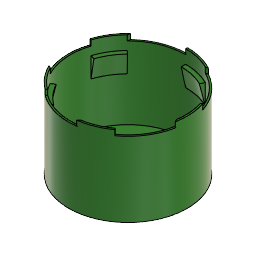
frame-base (Autodesk Fusion 360 design; units mm, degrees)
part number: 2026-06-05-14-14-42-148
Autodesk Fusion 360 part; units mm, degrees
note: some values were not read from the file. Set by a fixed rule: which sketch regions a step uses.
sketch "Sketch1" plane through (0, 0, 0) normal (0, 0, 1) x (1, 0, 0)
  circle A0 centre (0, 0) radius 65.5
  circle A1 centre (0, 0) radius 67.5
  line L0 (0, 0) -> (0, 65.5)
  line L1 (0, 0) -> (29.226, 58.6182)
  line L2 (29.226, 58.6182) -> (32.4791, 59.1723)
  line L3 (0, 65.5) -> (0, 67.5)
  line L4 (-62.2942, 20.2406) -> (-64.1963, 20.8586)
  line L5 (-46.7179, 45.9096) -> (-46.2396, 49.1747)
  line L6 (-38.4999, -52.9906) -> (-39.6755, -54.6086)
  line L7 (-58.0992, -30.2445) -> (-61.0567, -28.7806)
  line L8 (38.4999, -52.9906) -> (39.6755, -54.6086)
  line L9 (10.8106, -64.6017) -> (8.5044, -66.9621)
  line L10 (62.2942, 20.2406) -> (64.1963, 20.8586)
  line L11 (64.7805, -9.6815) -> (66.3128, -12.6042)
  line L12 (0, 60.5) -> (0, 65.5)
  line L13 (26.995, 54.1435) -> (29.226, 58.6182)
  arc A2 (26.995, 54.1435) -> (0, 60.5) centre (0, 0) ccw
  line L14 (-57.5389, 18.6955) -> (-62.2942, 20.2406)
  arc A3 (-43.1517, 42.405) -> (-57.5389, 18.6955) centre (0, 0) ccw
  line L15 (-43.1517, 42.405) -> (-46.7179, 45.9096)
  line L16 (-35.561, -48.9455) -> (-38.4999, -52.9906)
  arc A4 (-53.6642, -27.9358) -> (-35.561, -48.9455) centre (0, 0) ccw
  line L17 (-53.6642, -27.9358) -> (-58.0992, -30.2445)
  line L18 (35.561, -48.9455) -> (38.4999, -52.9906)
  arc A5 (9.9854, -59.6703) -> (35.561, -48.9455) centre (0, 0) ccw
  line L19 (9.9854, -59.6703) -> (10.8106, -64.6017)
  line L20 (57.5389, 18.6955) -> (62.2942, 20.2406)
  arc A6 (59.8355, -8.9425) -> (57.5389, 18.6955) centre (0, 0) ccw
  line L21 (59.8355, -8.9425) -> (64.7805, -9.6815)
  dimension "d1" = 131
  dimension "d2" = 135
  dimension "d3" = 26.5
  dimension "d4" = 3.3
  dimension "d8" = 360
  dimension "d13" = 121
  dimension "d15" = 360
  constraint coincident A0.centre A1.centre
  constraint concentric A0 A1
  constraint vertical L0
  constraint coincident A0 L1.end
  constraint coincident A0 L0.end
  constraint coincident A1 L2.end
  constraint coincident A1 L3.end
  constraint parallel L0 L3
  constraint concentric A0 A2
  constraint coincident L0 L12.start
  constraint coincident L1 L13.start
  measures "d1" diameter of A0
  measures "d2" diameter of A1
  measures "d3" angle of L0 L1
  measures "d4" distance of L1.end L2.end
  measures "d13" diameter of A2
extrude "Extrude1" add sketch "Sketch1" along normal blind 2.5 contours A0 L20 A6 L21 | A0 L0 L1 L12 L13 L14 A3 L15 L16 A4 L17 L18 A5 L19 L20 A6 L21 | A0 L0 L1 L12 L13 A2 | A0 L18 A5 L19 | L0 L1 A2 | A0 L14 A3 L15 | A0 L16 A4 L17 makes body 1
extrude "Extrude2" add sketch "Sketch1" along normal blind 85 contours A0 A1 L2 L10 | A0 A1 L8 L11 | A0 A1 L3 L5 | A0 A1 L6 L9 | A0 A1 L4 L7 bodies 1
extrude "Extrude3" add sketch "Sketch1" along normal blind 91 contours A0 A1 L10 L11 | A0 A1 L2 L3 | A0 A1 L8 L9 | A0 A1 L4 L5 | A0 A1 L6 L7 bodies 1
extrude "Extrude4" add sketch "Sketch1" along normal blind 23 from surface at 52.5 separate body contours A0 L20 A6 L21 | A0 L0 L1 L12 L13 A2 | A0 L18 A5 L19 | A0 L14 A3 L15 | A0 L16 A4 L17 makes body 2 at (-40.5132, -51.4677, 67.8333) makes body 3 at (-48.4522, 44.0753, 67.8333) makes body 4 at (22.9832, -61.3353, 67.8333) makes body 5 at (2.5239, 65.4514, 67.8333) makes body 6 at (65.3337, -4.6641, 67.8333)
sketch "Sketch2" plane through (0, 0, 0) normal (-0.147809, -0.989016, 0) x (0.989016, -0.147809, 0)
  line L0 (60.5, 52.5) -> (65.5, 52.5)
  line L1 (65.5, 52.5) -> (65.5, 75.5)
  line L2 (65.5, 75.5) -> (60.5, 75.5)
  line L3 (60.5, 75.5) -> (60.5, 52.5)
  line L4 (60.5, 75.5) -> (65.5, 52.5)
  constraint coincident L2.end L3.start
  constraint coincident L0.end L1.start
revolve "Revolve1" cut sketch "Sketch2" angle 360 about axis through (0, 0, 1.75) along (0, 0, 1) contours L0 L3 L4 bodies 2 3 4 5 6
equation "d1 = ( 65.5 * 2 ) * 1 mm"
equation "d2 = ( 67.5 * 2 ) * 1 mm"
